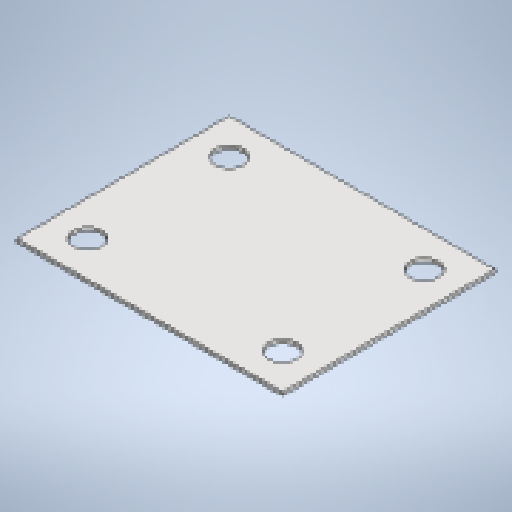
# Autodesk Inventor part: Part2
Saved by Autodesk Inventor 2025 (Build 290162010, 162A)
## iProperties
Created: 2025-11-03
Part Number: Part2
Material: Generic
Description: DIE16(5)|\ 90°|corrY -___°|X_____|bom___
Document SubType Name: Sheet Metal
Designer: admin
Stock Number: МОО 305 шпангоут борт
Mass: 1762.25 g
Surface Area: 2283.33 cm^2
Volume: 220.281 cm^3
Density: 1 g/cm^3
Sheet Metal Rule: Default
Sheet Metal Width: 0.000 mm
Sheet Metal Length: 0.000 mm
Sheet Metal Area: 0.000 mm^2
Appearance: Default
Author: admin
Autodesk Inventor part; units mm, degrees
ref_plane "YZ Plane" through (0, 0, 0) normal (1, 0, 0) x (0, 1, 0)
ref_plane "XZ Plane" through (0, 0, 0) normal (0, 1, 0) x (-1, 0, 0)
ref_plane "XY Plane" through (0, 0, 0) normal (0, 0, 1) x (1, 0, 0)
sketch "Sketch1" plane through (0, 0, 0) normal (0, 0, 1) x (1, 0, 0)
  line L0 (-80, -100) -> (80, -100)
  line L1 (80, -100) -> (80, 100)
  line L2 (80, 100) -> (-80, 100)
  line L3 (-80, 100) -> (-80, -100)
  line L4 (-80, -100) -> (80, 100) construction
  line L5 (80, -100) -> (-80, 100) construction
  circle A0 centre (-60, 80) radius 8
  circle A1 centre (-60, -80) radius 8
  circle A2 centre (60, 80) radius 8
  circle A3 centre (60, -80) radius 8
  line L6 (0, 100) -> (0, -100) construction
  line L7 (-80, 0) -> (80, 0) construction
  point P0 (0, 0)
  dimension "d154" = 160
  dimension "d155" = 200
  dimension "d157" = 20
  dimension "d158" = 20
  dimension "d159" = 16
  dimension "d161" = 160
  measures "d154" distance of L1.end L2.end
  measures "d155" distance of L0.end L1.end
  measures "d157" distance from line of L2 A0.centre
  measures "d158" distance from line of L3 A0.centre
  measures "d159" diameter of A0
  measures "d161" distance of A3.centre A2.centre
extrude "Plate5" add sketch "Sketch1" along normal blind 6
fillet "Corner Round1" radius 6 4 edges at (-80, 100, 3) (80, 100, 3) (80, -100, 3) (-80, -100, 3)
body "Solid3"
